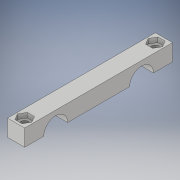
# Autodesk Inventor part: Mount_Block
Saved by Autodesk Inventor 2019 (Build 230136000, 136)
## iProperties
Created: 2019-10-21
Part Number: Mount_Block
Material: Generic
Document SubType Name: Modeling
Designer: 19879326
Density: 1 g/cm^3
Appearance: Default
Author: 19879326
Autodesk Inventor part; units mm, degrees
ref_plane "YZ Plane" through (0, 0, 0) normal (1, 0, 0) x (0, 1, 0)
ref_plane "XZ Plane" through (0, 0, 0) normal (0, 1, 0) x (-1, 0, 0)
ref_plane "XY Plane" through (0, 0, 0) normal (0, 0, 1) x (1, 0, 0)
sketch "Sketch1" plane through (0, 0, 0) normal (1, 0, 0) x (0, 1, 0)
  arc A0 (0, 32.5) -> (0, 57.5) centre (0, 45) ccw
  arc A1 (0, -57.5) -> (0, -32.5) centre (0, -45) ccw
  line L0 (0, 77.5) -> (17.5, 77.5)
  line L1 (17.5, 77.5) -> (17.5, -77.5)
  line L2 (17.5, -77.5) -> (0, -77.5)
  line L3 (0, 57.5) -> (0, 77.5)
  line L4 (0, -77.5) -> (0, -57.5)
  line L5 (0, -32.5) -> (0, 32.5)
  point P0 (0, 0)
  point P1 (0, 0)
  point P2 (17.5, 0)
  point P3 (0, 67.5)
  point P4 (0, -67.5)
  point P5 (12.5, 45)
  dimension "d0" = 25
  dimension "d2" = 90
  dimension "d3" = 45
  dimension "d4" = 20
  dimension "d15" = 5
  constraints: 12 end point, 5 point on circle, 4 midpoint, 4 parallel, 3 vertical alignment, 2 centre point, 2 coincident, 1 equal radius, 1 horizontal, 1 horizontal alignment, 1 perpendicular
  measures "d0" diameter of A0
  measures "d2" distance of A1.centre A0.centre
  measures "d3" distance of point (0, 0) A1.centre
  measures "d4" distance from line of L0 L3.start
  measures "d15" distance from line of L1 point (12.5, 45)
extrude "Extrusion1" add sketch "Sketch1" along normal blind 18
sketch "Sketch2" plane through (0, 17.5, 77.5) normal (0, 1, 0) x (1, 0, 0)
  circle A0 centre (9, 9) radius 4
  circle A1 centre (9, 146) radius 4
  line L0 (18, 155) -> (18, 0) projected
  line L1 (0, 0) -> (18, 0) projected
  line L2 (0, 155) -> (18, 155) projected
  point P0 (0, 77.5)
  dimension "d7" = 8
  dimension "d8" = 8
  dimension "d9" = 9
  dimension "d10" = 9
  dimension "d11" = 9
  constraints: 2 centre point, 1 vertical alignment
  measures "d7" diameter of A0
  measures "d8" diameter of A1
  measures "d9" distance from line of L0 A0.centre
  measures "d10" distance from line of A0.centre L1
  measures "d11" distance from line of L2 A1.centre
extrude "Extrusion2" cut sketch "Sketch2" against normal blind 29.5
sketch "Sketch3" plane through (0, 17.5, 77.5) normal (0, 1, 0) x (1, 0, 0)
  circle A0 centre (9, 146) radius 4 projected
  line L0 (12.7528, 152.5) -> (16.5056, 146)
  line L1 (16.5056, 146) -> (12.7528, 139.5)
  line L2 (12.7528, 139.5) -> (5.2472, 139.5)
  line L3 (5.2472, 139.5) -> (1.4944, 146)
  line L4 (1.4944, 146) -> (5.2472, 152.5)
  line L5 (5.2472, 152.5) -> (12.7528, 152.5)
  line L6 (0, 155) -> (18, 155) projected
  circle A1 centre (9, 9) radius 4 projected
  line L7 (12.7528, 2.5) -> (5.2472, 2.5)
  line L8 (5.2472, 2.5) -> (1.4944, 9)
  line L9 (1.4944, 9) -> (5.2472, 15.5)
  line L10 (5.2472, 15.5) -> (12.7528, 15.5)
  line L11 (12.7528, 15.5) -> (16.5056, 9)
  line L12 (16.5056, 9) -> (12.7528, 2.5)
  line L13 (0, 0) -> (18, 0) projected
  point P0 (0, 77.5)
  dimension "d16" = 13
  dimension "d17" = 13
  constraints: 24 end point, 2 coincident, 2 parallel, 26 other
  measures "d16" distance between parallel lines of L2 L5
  measures "d17" distance between parallel lines of L10 L7
extrude "Extrusion3" cut sketch "Sketch3" against normal blind 5
body "Solid1"
